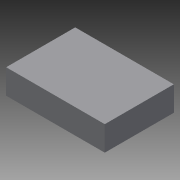
# Autodesk Inventor part: power board
Saved by Autodesk Inventor 2015 (Build 190159000, 159)
## iProperties
Created: 2014-10-23
Part Number: power board
Material: Generic
Document SubType Name: Modeling
Designer: ericd_000
Density: 1 g/cm^3
Appearance: Default
Author: ericd_000
Autodesk Inventor part; units mm, degrees
ref_plane "YZ Plane" through (0, 0, 0) normal (1, 0, 0) x (0, 1, 0)
ref_plane "XZ Plane" through (0, 0, 0) normal (0, 1, 0) x (-1, 0, 0)
ref_plane "XY Plane" through (0, 0, 0) normal (0, 0, 1) x (1, 0, 0)
sketch "Sketch1" plane through (0, 0, 0) normal (0, 0, 1) x (1, 0, 0)
  line L0 (-12.1136, 8.8959) -> (27.8864, 8.8959)
  line L1 (27.8864, 8.8959) -> (27.8864, -19.1167)
  line L2 (27.8864, -19.1167) -> (-12.1136, -19.1167)
  line L3 (-12.1136, -19.1167) -> (-12.1136, 8.8959)
  point P0 (0, 0)
  dimension "d0" = 40
  constraints: 8 end point, 2 parallel, 1 horizontal, 1 perpendicular
  measures "d0" distance of L0.start L0.end
extrude "Extrusion1" add sketch "Sketch1" along normal blind 10
body "Solid1"
